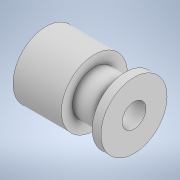
# Autodesk Inventor part: IdlerPulley
Saved by Autodesk Inventor 2022 (Build 260153000, 153)
## iProperties
Created: 2021-06-16
Part Number: IdlerPulley
Material: Generic
Document SubType Name: Modeling
Designer: burgessb
Density: 1 g/cm^3
Appearance: Default
Author: burgessb
Autodesk Inventor part; units mm, degrees
ref_plane "YZ Plane" through (0, 0, 0) normal (1, 0, 0) x (0, 1, 0)
ref_plane "XZ Plane" through (0, 0, 0) normal (0, 1, 0) x (-1, 0, 0)
ref_plane "XY Plane" through (0, 0, 0) normal (0, 0, 1) x (1, 0, 0)
sketch "Sketch1" plane through (0, 0, 0) normal (0, 1, 0) x (-1, 0, 0)
  line L0 (0, 0) -> (0, -7.5)
  line L1 (0, -7.5) -> (2, -7.5)
  line L2 (2, -7.5) -> (2, -5)
  line L3 (2, -5) -> (9, -5)
  line L4 (9, -5) -> (9, -7.5)
  line L5 (9, -7.5) -> (20, -7.5)
  line L6 (20, -7.5) -> (20, 0)
  line L7 (20, 0) -> (0, 0)
  line L8 (0, -2.7) -> (20, -2.7)
  dimension "d0" = 7.5
  dimension "d1" = 7.5
  dimension "d2" = 5
  dimension "d3" = 2
  dimension "d4" = 11
  dimension "d5" = 7
  dimension "d7" = 2.7
  constraints: 18 end point, 6 perpendicular, 4 point on line, 1 vertical
  measures "d0" distance of L0.start L0.end
  measures "d1" distance of L5.end L6.end
  measures "d2" distance from line of L0.start L3
  measures "d3" distance between parallel lines of L0 L2
  measures "d4" distance of L4.end L5.end
  measures "d5" distance of L2.end L3.end
  measures "d7" distance from line of L0.start L8
revolve "Revolution1" add sketch "Sketch1" angle 360 about axis through (-20, 0, 0) along (1, 0, 0) contours L8 L6 L5 L4 L3 L2 L1 L0
equation "\"d1\" = d0"
body "Solid1"
